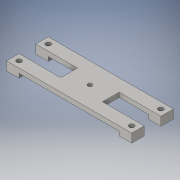
# Autodesk Inventor part: Camera Mount
Saved by Autodesk Inventor 2016 (Build 200138000, 138)
## iProperties
Created: 2017-10-12
Part Number: Camera Mount
Material: Generic
Document SubType Name: Modeling
Designer: Student
Density: 1 g/cm^3
Appearance: Default
Author: Student
Autodesk Inventor part; units mm, degrees
ref_plane "YZ Plane" through (0, 0, 0) normal (1, 0, 0) x (0, 1, 0)
ref_plane "XZ Plane" through (0, 0, 0) normal (0, 1, 0) x (-1, 0, 0)
ref_plane "XY Plane" through (0, 0, 0) normal (0, 0, 1) x (1, 0, 0)
sketch "Sketch1" plane through (0, 0, 0) normal (0, 1, 0) x (-1, 0, 0)
  line L0 (8.5745, -14.965) -> (8.5745, 10.435)
  line L1 (8.5745, 10.435) -> (-16.8255, 10.435)
  line L2 (-16.8255, 10.435) -> (-16.8255, -14.965)
  line L3 (-16.8255, -14.965) -> (8.5745, -14.965)
  point P0 (0, 0)
  dimension "d0" = 25.4
  dimension "d1" = 25.4
  constraints: 8 end point, 3 perpendicular, 1 vertical
  measures "d0" distance of L0.start L0.end
  measures "d1" distance of L2.end L0.start
extrude "Extrusion1" add sketch "Sketch1" along normal blind 2.794
sketch "Sketch2" plane through (16.8255, 0, 10.435) normal (1, 0, 0) x (0, 0, -1)
  line L0 (25.4, 2.794) -> (0, 2.794) projected
  line L1 (25.4, 0) -> (0, 0) projected
  line L2 (0, 2.794) -> (7.62, 2.794)
  line L3 (7.62, 2.794) -> (7.62, 0)
  line L4 (7.62, 0) -> (0, 0)
  line L5 (0, 0) -> (0, 2.794)
  line L6 (25.4, 0) -> (17.78, 0)
  line L7 (17.78, 0) -> (17.78, 2.794)
  line L8 (17.78, 2.794) -> (25.4, 2.794)
  line L9 (25.4, 2.794) -> (25.4, 0)
  point P0 (10.435, 0)
  dimension "d4" = 7.62
  dimension "d5" = 7.62
  constraints: 16 end point, 4 parallel, 2 horizontal, 2 perpendicular, 2 point on line
  measures "d4" distance of L7.end L8.end
  measures "d5" distance of L0.end L2.end
extrude "Extrusion2" add sketch "Sketch2" along normal blind 25.4 and the other way blind 50.8 contours L9 L1 L7 L0 | L3 L1 L5 L0
sketch "Sketch3" plane through (0, 0, 0) normal (0, -1, 0) x (1, 0, 0)
  line L0 (16.8255, 2.815) -> (16.8255, -7.345) construction
  line L1 (16.8255, -2.265) -> (-8.5745, -2.265) construction
  line L2 (-8.5745, -7.345) -> (-8.5745, 2.815) construction
  line L3 (42.2255, -14.965) -> (-33.9745, -14.965) construction
  line L4 (4.1255, -14.965) -> (4.1255, 10.435) construction
  line L5 (-33.9745, 10.435) -> (42.2255, 10.435) construction
  circle A0 centre (4.1255, -2.265) radius 1.27
  point P0 (0, 0)
  dimension "d10" = 2.54
  constraints: 5 midpoint, 4 end point, 1 centre point
  measures "d10" diameter of A0
extrude "Extrusion3" cut sketch "Sketch3" against normal blind 25.4
sketch "Sketch4" plane through (0, 0, 0) normal (0, -1, 0) x (1, 0, 0)
  line L0 (-33.9745, -14.965) -> (42.2255, -14.965) projected
  line L1 (16.8255, -7.345) -> (42.2255, -7.345) projected
  line L2 (42.2255, -14.965) -> (34.6055, -14.965)
  line L3 (34.6055, -14.965) -> (34.6055, -7.345)
  line L4 (34.6055, -7.345) -> (42.2255, -7.345)
  line L5 (42.2255, -7.345) -> (42.2255, -14.965)
  line L6 (42.2255, 10.435) -> (-33.9745, 10.435) projected
  line L7 (-33.9745, -7.345) -> (-33.9745, -14.965) projected
  line L8 (-33.9745, -7.345) -> (-8.5745, -7.345) projected
  line L9 (-33.9745, -14.965) -> (-26.3545, -14.965)
  line L10 (-26.3545, -14.965) -> (-26.3545, -7.345)
  line L11 (-26.3545, -7.345) -> (-33.9745, -7.345)
  line L12 (-33.9745, -7.345) -> (-33.9745, -14.965)
  line L13 (-33.9745, 10.435) -> (-33.9745, 2.815) projected
  line L14 (-33.9745, 2.815) -> (-26.3545, 2.815)
  line L15 (-26.3545, 2.815) -> (-26.3545, 10.435)
  line L16 (-26.3545, 10.435) -> (-33.9745, 10.435)
  line L17 (-33.9745, 10.435) -> (-33.9745, 2.815)
  line L18 (42.2255, 2.815) -> (42.2255, 10.435) projected
  line L19 (-33.9745, 10.435) -> (42.2255, 10.435) projected
  line L20 (42.2255, 2.815) -> (34.6055, 2.815)
  line L21 (34.6055, 2.815) -> (34.6055, 10.435)
  line L22 (34.6055, 10.435) -> (42.2255, 10.435)
  line L23 (42.2255, 10.435) -> (42.2255, 2.815)
  point P0 (0, 0)
  dimension "d13" = 7.62
  dimension "d14" = 7.62
  dimension "d15" = 7.62
  constraints: 32 end point, 8 parallel, 4 horizontal, 4 perpendicular, 4 point on line
  measures "d13" distance of L0.start L9.end
  measures "d14" distance of L13.end L14.end
  measures "d15" distance of L0.end L2.end
extrude "Extrusion4" add sketch "Sketch4" along normal blind 2.54
sketch "Sketch5" plane through (0, -2.54, 0) normal (0, -1, 0) x (1, 0, 0)
  line L0 (42.2255, -14.965) -> (42.2255, -7.345) projected
  line L1 (34.6055, -14.965) -> (34.6055, -7.345) projected
  line L2 (42.2255, -14.965) -> (34.6055, -14.965)
  line L3 (34.6055, -14.965) -> (34.6055, -7.345)
  line L4 (34.6055, -7.345) -> (42.2255, -7.345)
  line L5 (42.2255, -7.345) -> (42.2255, -14.965)
  circle A0 centre (38.4155, -11.155) radius 1.5
  circle A1 centre (38.4155, 6.625) radius 1.5012
  line L6 (34.6055, 10.435) -> (34.6055, 2.815) projected
  circle A2 centre (-30.1645, 6.625) radius 1.5
  line L7 (-33.9745, 2.815) -> (-26.3545, 2.815) projected
  circle A3 centre (-30.1645, -11.155) radius 1.5
  point P0 (0, 0)
  point P1 (34.6055, 6.625)
  point P2 (-30.1645, 2.815)
  dimension "d18" = 3
  dimension "d19" = 3
  dimension "d20" = 3.0024
  dimension "d21" = 3
  constraints: 8 end point, 4 centre point, 2 midpoint, 2 parallel, 1 horizontal, 1 horizontal alignment, 1 perpendicular, 1 vertical alignment
  measures "d18" diameter of A0
  measures "d19" diameter of A2
  measures "d20" diameter of A1
  measures "d21" diameter of A3
extrude "Extrusion5" cut sketch "Sketch5" against normal blind 76.2 contours A0 | A1 | A2 | A3
equation "\"d5\" = d4"
body "Solid1"
